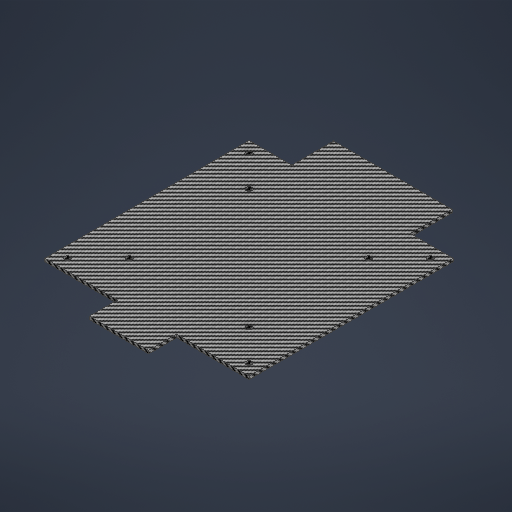
# Autodesk Inventor part: swtc2
Saved by Autodesk Inventor 2026.1 (Build 301233020, 233B)
## iProperties
Created: 2025-07-24
Part Number: swtc2
Material: Polímero reforzado con fibra de carbono
Document SubType Name: Modeling
Designer: rodri
Density: 1.43 g/cm^3
Appearance: Fibra de carbono
Author: rodri
Autodesk Inventor part; units mm, degrees
ref_plane "YZ Plane" through (0, 0, 0) normal (1, 0, 0) x (0, 1, 0)
ref_plane "XZ Plane" through (0, 0, 0) normal (0, 1, 0) x (-1, 0, 0)
ref_plane "XY Plane" through (0, 0, 0) normal (0, 0, 1) x (1, 0, 0)
sketch "Boceto4" plane through (0, 0, 0) normal (0, 1, 0) x (-1, 0, 0)
  line L0 (-58.5, -58.5) -> (58.5, -58.5)
  line L1 (58.5, -58.5) -> (58.5, 58.5)
  line L2 (58.5, 58.5) -> (-58.5, 58.5)
  line L3 (-58.5, 58.5) -> (-58.5, -58.5)
  line L4 (-58.5, -58.5) -> (58.5, 58.5) construction
  line L5 (58.5, -58.5) -> (-58.5, 58.5) construction
  line L6 (-52, 52) -> (52, 52) construction
  line L7 (52, 52) -> (52, -52) construction
  line L8 (52, -52) -> (-52, -52) construction
  line L9 (-52, -52) -> (-52, 52) construction
  line L10 (-52, 52) -> (52, -52) construction
  line L11 (52, 52) -> (-52, -52) construction
  line L12 (-34.3223, -34.3223) -> (34.3223, -34.3223) construction
  line L13 (34.3223, -34.3223) -> (34.3223, 34.3223) construction
  line L14 (34.3223, 34.3223) -> (-34.3223, 34.3223) construction
  line L15 (-34.3223, 34.3223) -> (-34.3223, -34.3223) construction
  line L16 (-34.3223, -34.3223) -> (34.3223, 34.3223) construction
  line L17 (34.3223, -34.3223) -> (-34.3223, 34.3223) construction
  line L18 (0, -58.5) -> (0, -82.5) construction
  line L19 (34, -58.5) -> (-34, -58.5)
  line L20 (-34, -58.5) -> (-34, -82.5)
  line L21 (-34, -82.5) -> (34, -82.5)
  line L22 (34, -82.5) -> (34, -58.5)
  line L23 (34, -58.5) -> (-34, -82.5) construction
  line L24 (-34, -58.5) -> (34, -82.5) construction
  line L25 (0, 58.5) -> (0, 74.5) construction
  line L26 (17, 58.5) -> (-17, 58.5)
  line L27 (-17, 58.5) -> (-17, 74.5)
  line L28 (-17, 74.5) -> (17, 74.5)
  line L29 (17, 74.5) -> (17, 58.5)
  line L30 (17, 58.5) -> (-17, 74.5) construction
  line L31 (-17, 58.5) -> (17, 74.5) construction
  point P0 (0, 0)
  point P1 (0, -70.5)
  point P2 (0, 66.5)
  dimension "d35" = 117
  dimension "d36" = 117
  dimension "d37" = 104
  dimension "d38" = 104
  dimension "d39" = 25
  dimension "d49" = 24
  dimension "d50" = 68
  dimension "d51" = 16
  dimension "d52" = 34
  constraints: 64 end point, 14 midpoint, 10 parallel, 5 horizontal, 5 perpendicular, 2 vertical, 1 point on line
  measures "d35" distance of L0.start L0.end
  measures "d36" distance of L0.end L1.end
  measures "d37" distance of L7.end L8.end
  measures "d38" distance of L6.end L7.end
  measures "d39" distance of L13.end L6.end
  measures "d49" distance of L18.start L18.end
  measures "d50" distance of L20.end L21.end
  measures "d51" distance of L25.start L25.end
  measures "d52" distance of L27.end L28.end
extrude "Extrusión3" add sketch "Boceto4" against normal blind 1.8
hole "Agujero2" at (-52, 0, -52) at (52, 0, -52) at (34.3223, 0, -34.3223) at (-34.3223, 0, -34.3223) at (-52, 0, 52) at (-34.3223, 0, 34.3223) at (52, 0, 52) at (34.3223, 0, 34.3223) direction (0, -1, 0) diameter 3.4 end through all clearance for "Tornillo para maquinaria de cabeza plana" size "M3" standard "Perfil M métrico ANSI"
